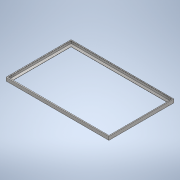
# Autodesk Inventor part: frame
Saved by Autodesk Inventor 2020 (Build 240168000, 168)
## iProperties
Created: 2020-06-26
Part Number: frame
Material: Generic
Document SubType Name: Modeling
Designer: Abbas
Density: 1 g/cm^3
Appearance: Default
Author: Abbas
Autodesk Inventor part; units mm, degrees
ref_plane "YZ Plane" through (0, 0, 0) normal (1, 0, 0) x (0, 1, 0)
ref_plane "XZ Plane" through (0, 0, 0) normal (0, 1, 0) x (-1, 0, 0)
ref_plane "XY Plane" through (0, 0, 0) normal (0, 0, 1) x (1, 0, 0)
sketch "Sketch1" plane through (0, 0, 0) normal (0, 1, 0) x (-1, 0, 0)
  line L0 (533, 337) -> (-533, 337)
  line L1 (-533, 337) -> (-533, -337)
  line L2 (-533, -337) -> (533, -337)
  line L3 (533, -337) -> (533, 337)
  line L4 (533, 337) -> (-533, -337) construction
  line L5 (-533, 337) -> (533, -337) construction
  line L6 (531, 335) -> (-531, 335)
  line L7 (-531, 335) -> (-531, -335)
  line L8 (-531, -335) -> (531, -335)
  line L9 (531, -335) -> (531, 335)
  line L10 (531, 335) -> (-531, -335) construction
  line L11 (-531, 335) -> (531, -335) construction
  line L12 (503, 307) -> (-503, 307)
  line L13 (-503, 307) -> (-503, -307)
  line L14 (-503, -307) -> (503, -307)
  line L15 (503, -307) -> (503, 307)
  line L16 (503, 307) -> (-503, -307) construction
  line L17 (-503, 307) -> (503, -307) construction
  point P0 (0, 0)
  dimension "d0" = 1066
  dimension "d1" = 674
  dimension "d2" = 1062
  dimension "d3" = 670
  dimension "d4" = 1006
  dimension "d5" = 614
  constraints: 36 end point, 6 midpoint, 6 parallel, 3 horizontal, 3 perpendicular
  measures "d0" distance of L2.end L1.end
  measures "d1" distance of L1.end L0.end
  measures "d2" distance of L8.end L7.end
  measures "d3" distance of L7.end L6.end
  measures "d4" distance of L14.end L13.end
  measures "d5" distance of L13.end L12.end
extrude "Extrusion1" add sketch "Sketch1" along normal blind 2 contours L9 L8 L7 L6
extrude "Extrusion2" add sketch "Sketch1" along normal blind 33 contours L3 L2 L1 L0
sketch "Sketch2" plane through (0, 33, 0) normal (0, 1, 0) x (1, 0, 0)
  line L0 (-533, -337) -> (533, -337)
  line L1 (533, -337) -> (533, 337)
  line L2 (533, 337) -> (-533, 337)
  line L3 (-533, 337) -> (-533, -337)
  line L4 (-533, -337) -> (533, 337) construction
  line L5 (533, -337) -> (-533, 337) construction
  line L6 (-523, -327) -> (523, -327)
  line L7 (523, -327) -> (523, 327)
  line L8 (523, 327) -> (-523, 327)
  line L9 (-523, 327) -> (-523, -327)
  line L10 (-523, -327) -> (523, 327) construction
  line L11 (523, -327) -> (-523, 327) construction
  point P0 (0, 0)
  dimension "d10" = 1066
  dimension "d11" = 674
  dimension "d12" = 1046
  dimension "d13" = 654
  constraints: 24 end point, 4 midpoint, 4 parallel, 2 horizontal, 2 perpendicular
  measures "d10" distance of L2.end L1.end
  measures "d11" distance of L1.end L0.end
  measures "d12" distance of L8.end L7.end
  measures "d13" distance of L7.end L6.end
extrude "Extrusion3" add sketch "Sketch2" along normal blind 2
body "Solid1"
